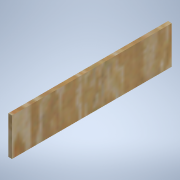
# Autodesk Inventor part: Front
Saved by Autodesk Inventor 2021.1 (Build 251245000, 245)
## iProperties
Created: 2020-08-02
Part Number: Front
Material: Generic
Document SubType Name: Modeling
Designer: adick
Density: 1 g/cm^3
Appearance: Default
Author: adick
Autodesk Inventor part; units mm, degrees
ref_plane "YZ Plane" through (0, 0, 0) normal (1, 0, 0) x (0, 1, 0)
ref_plane "XZ Plane" through (0, 0, 0) normal (0, 1, 0) x (-1, 0, 0)
ref_plane "XY Plane" through (0, 0, 0) normal (0, 0, 1) x (1, 0, 0)
sketch "Sketch1" plane through (0, 0, 0) normal (0, 0, 1) x (1, 0, 0)
  line L0 (135, -70.65) -> (-135, -70.65) projected
  line L1 (-135, -7) -> (-128.65, -7)
  line L2 (-128.65, -7) -> (-128.65, -70.65)
  line L3 (-128.65, -70.65) -> (-135, -70.65)
  line L4 (-135, -70.65) -> (-135, -7)
  point P0 (0, 0)
  dimension "d0" = 6.35
  constraints: 8 end point, 2 parallel, 1 horizontal, 1 perpendicular, 1 point on line, 1 other
  measures "d0" distance of L2.end L3.end
extrude "Extrusion1" add sketch "Sketch1" along normal blind 270
body "Solid1"
